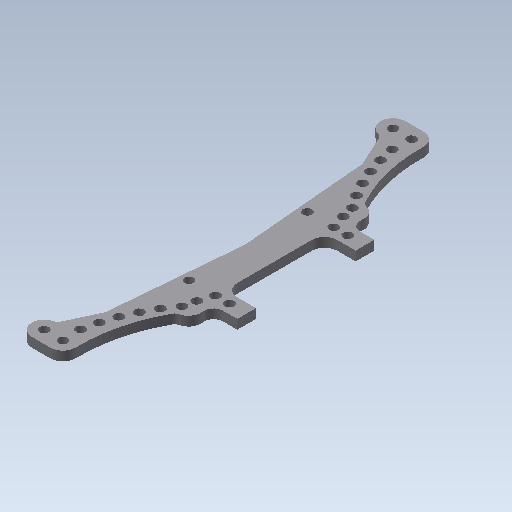
# Autodesk Inventor part: 500-120
Saved by Autodesk Inventor 2020 (Build 240168000, 168)
## iProperties
Created: 2015-04-18
Part Number: 500-120
Material: Generic
Document SubType Name: Modeling
Designer: Station9
Density: 1 g/cm^3
Appearance: Default
Mass: 3.63984 g
Surface Area: 40.1543 cm^2
Volume: 3.63984 cm^3
Author: Station9
Autodesk Inventor part; units mm, degrees
ref_plane "YZ Plane" through (0, 0, 0) normal (1, 0, 0) x (0, 1, 0)
ref_plane "XZ Plane" through (0, 0, 0) normal (0, 1, 0) x (-1, 0, 0)
ref_plane "XY Plane" through (0, 0, 0) normal (0, 0, 1) x (1, 0, 0)
sketch "Sketch1" plane through (0, 0, 0) normal (0, 1, 0) x (-1, 0, 0)
  line L0 (0, -16) -> (0, -22)
  line L1 (0, -22) -> (4.5992, -22)
  arc A0 (7.5587, -25.4914) -> (4.5992, -22) centre (4.5992, -25) ccw
  arc A1 (7.5587, -25.4914) -> (10.6423, -30.0525) centre (11.5046, -26.1465) ccw
  arc A2 (18.0009, -55.917) -> (11.9694, -31.0524) centre (-31.9884, -54.8791) ccw
  arc A3 (18.0009, -55.917) -> (22, -60) centre (22, -56) ccw
  line L2 (22, -60) -> (28, -60)
  arc A4 (28, -60) -> (28.9223, -52.1078) centre (28, -56) ccw
  line L3 (27.5709, -51.0069) -> (23.1874, -41.6064)
  line L4 (23.0076, -40.9355) -> (19.4262, 0)
  arc A5 (11.9694, -31.0524) -> (10.6423, -30.0525) centre (10.2111, -32.0054) ccw
  line L5 (0, -16) -> (6, -16)
  line L6 (10, -12) -> (10, 0)
  arc A6 (6, -16) -> (10, -12) centre (6, -12) ccw
  arc A7 (22.2903, -50.042) -> (12.4, -27.35) centre (-30.8395, -59.6973) ccw
  line L7 (28, -56) -> (42.0245, -56)
  line L8 (22.2903, -50.042) -> (35.4778, -47.6454)
  line L9 (-30.8395, -59.6973) -> (22.2903, -50.042)
  line L10 (-30.8395, -59.6973) -> (12.4, -27.35)
  circle A8 centre (22.2903, -50.042) radius 1.5
  circle A9 centre (21.1713, -45.1756) radius 1.5
  circle A10 centre (19.6075, -40.4334) radius 1.5
  circle A11 centre (17.6125, -35.856) radius 1.5
  circle A12 centre (15.2031, -31.4824) radius 1.5
  circle A13 centre (12.4, -27.35) radius 1.5
  circle A14 centre (5.5, -19) radius 1.5
  circle A15 centre (10, -19) radius 1.5
  circle A16 centre (18.5, -19) radius 1.5
  circle A17 centre (11.5, -23.5) radius 1.5
  circle A18 centre (28, -56) radius 1.5
  circle A19 centre (22, -56) radius 1.5
  arc A20 (23.0076, -40.9355) -> (23.1874, -41.6064) centre (25, -40.7612) ccw
  arc A21 (27.5709, -51.0069) -> (28.9223, -52.1078) centre (29.3835, -50.1617) ccw
  line L11 (19.4262, 0) -> (10, 0)
  point P0 (0, 0)
  point P1 (28.0341, -52.0001)
  dimension "d0" = 28
  dimension "d1" = 0
  dimension "d2" = 2
  dimension "d3" = 4
  dimension "d4" = 12
  dimension "d5" = 0
  dimension "d6" = 10
  dimension "d8" = 5
  dimension "d9" = 20
  dimension "d10" = 4
  dimension "d11" = 4
  dimension "d12" = 50
  dimension "d13" = 4
  dimension "d14" = 3
  dimension "d15" = 54
  dimension "d16" = 10.3
  dimension "d17" = 26.5
  dimension "d18" = 27.35
  dimension "d19" = 12.4
  dimension "d20" = 3
  dimension "d21" = 56
  dimension "d22" = 0
  dimension "d25" = 26.5
  dimension "d28" = 3
  dimension "d29" = 3
  dimension "d30" = 3
  dimension "d31" = 5.5
  dimension "d32" = 4.5
  dimension "d34" = 19
  dimension "d35" = 3
  dimension "d36" = 4.5
  dimension "d38" = 13
  dimension "d39" = 3
  dimension "d40" = 6
  dimension "d42" = 3
  dimension "d43" = 3
  dimension "d44" = 2
  constraints: 24 end point, 22 point on circle, 21 centre point, 13 tangent, 3 coincident, 3 horizontal, 2 horizontal alignment, 2 perpendicular, 1 collinear, 1 equal radius, 1 point on line, 1 vertical, 14 other
  measures "d0" horizontal distance of point (0, 0) L7.start
  measures "d1" distance from line of point (0, 0) L0
  measures "d2" radius of A5
  measures "d3" radius of A6
  measures "d4" vertical distance of point (0, 0) A6.centre
  measures "d5" vertical distance of point (0, 0) L6.end
  measures "d6" distance between parallel lines of L0 L6
  measures "d8" angle of L6 L4
  measures "d9" angle of L4 L3
  measures "d10" radius of A4
  measures "d11" radius of A3
  measures "d12" radius of A2
  measures "d13" radius of A1
  measures "d14" radius of A0
  measures "d15" radius of A7
  measures "d16" angle of L7 L8
  measures "d17" angle of L9 L10
  measures "d18" vertical distance of point (0, 0) L10.end
  measures "d19" distance from line of L0 L10.end
  measures "d20" diameter of A8
  measures "d21" vertical distance of point (0, 0) L7.start
  measures "d22" vertical distance of point (0, 0) L4.end
  measures "d28" diameter of A14
  measures "d29" diameter of A15
  measures "d30" diameter of A16
  measures "d31" distance from line of L0 A14.centre
  measures "d32" distance of A15.centre A14.centre
  measures "d34" vertical distance of point (0, 0) A16.centre
  measures "d35" diameter of A17
  measures "d36" vertical distance of A16.centre A17.centre
  measures "d38" distance of A16.centre A14.centre
  measures "d39" distance from line of L1 A14.centre
  measures "d40" distance of L7.start A3.centre
  measures "d42" diameter of A18
  measures "d43" diameter of A19
  measures "d44" radius of A20
extrude "Extrusion2" add sketch "Sketch1" along normal blind 3 contours L5 A6 L6 L11 L4 A20 L3 L8 A8 A7 A9 A10 A11 A12 A13 L10 A1 A0 L1 L0 | L10 A13 A7 A12 A11 A10 A9 A8 L9 A2 A5 A1 | L9 A8 L8 L3 A21 A4 L2 A3 A2
mirror "Mirror1" about plane through (-19.4262, 0, 0) normal (0, 0, 1) of "Extrusion2"
body "Solid2"
